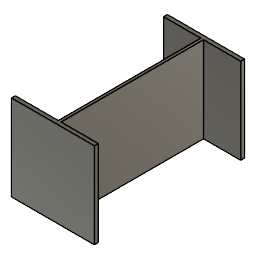
軽H-175×90×3.2×4.5 (Autodesk Fusion 360 design; units mm, degrees)
Autodesk Fusion 360 part; units mm, degrees
sketch "スケッチ1" plane through (0, 0, 0) normal (0, 0, 1) x (1, 0, 0)
  line L0 (0, -87.5) -> (0, 87.5)
  line L1 (-45, 87.5) -> (45, 87.5)
  line L2 (-51.735, -87.5) -> (-45, -87.5)
  line L3 (-45, -87.5) -> (45, -87.5)
  line L4 (-45, 83) -> (45, 83)
  line L5 (-51.735, -83) -> (-45, -83)
  line L6 (-45, -83) -> (45, -83)
  line L7 (1.6, -87.5) -> (1.6, 87.5)
  line L8 (-1.6, -87.5) -> (-1.6, 87.5)
  line L9 (-45, 87.5) -> (-45, 83)
  line L10 (45, 87.5) -> (45, 83)
  line L11 (45, -83) -> (45, -87.5)
  line L12 (-51.735, -83) -> (-51.735, -87.5)
  dimension "d1" = 175
  dimension "d2" = 90
  dimension "d3" = 90
  dimension "d4" = 4.5
  dimension "d5" = -4.5
  dimension "d6" = 1.6
  dimension "d7" = -1.6
  constraint vertical L0
  constraint midpoint origin L0
  constraint horizontal L1
  constraint midpoint L0.end L1
  constraint horizontal L2
  constraint parallel L2 L3
  constraint midpoint L0.start L3
  constraint perpendicular L4 L9
  constraint perpendicular L4 L10
  constraint perpendicular L6 L11
  constraint perpendicular L5 L12
  measures "d1" distance of L0.start L0.end
  measures "d2" distance of L1.start L1.end
  measures "d3" distance of L2.end L3.end
extrude "押し出し1" add sketch "スケッチ1" along normal blind 100
equation "d6 = ( 3.2 / 2 ) * 1 mm"
equation "d7 = ( -3.2 / 2 ) * 1 mm"
